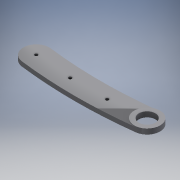
# Autodesk Inventor part: Arm 16X
Saved by Autodesk Inventor 2017 (Build 210142000, 142)
## iProperties
Created: 2016-03-22
Part Number: Arm 16X
Material: Generic
Document SubType Name: Modeling
Designer: alist
Density: 1 g/cm^3
Appearance: Default
Author: alist
Autodesk Inventor part; units mm, degrees
ref_plane "YZ Plane" through (0, 0, 0) normal (1, 0, 0) x (0, 1, 0)
ref_plane "XZ Plane" through (0, 0, 0) normal (0, 1, 0) x (-1, 0, 0)
ref_plane "XY Plane" through (0, 0, 0) normal (0, 0, 1) x (1, 0, 0)
sketch "Sketch1" plane through (0, 0, 0) normal (0, 0, 1) x (1, 0, 0)
  arc A0 (-74.2, 0) -> (74.2, 0) centre (0, 603.0231) ccw construction
  arc A1 (-76.3128, -17.1705) -> (76.3128, -17.1705) centre (0, 603.0231) ccw
  arc A2 (-72.0872, 17.1705) -> (72.0872, 17.1705) centre (0, 603.0231) ccw
  arc A3 (-72.0872, 17.1705) -> (-76.3128, -17.1705) centre (-74.2, 0) ccw
  arc A4 (76.3128, -17.1705) -> (72.0872, 17.1705) centre (74.2, 0) ccw
  line L0 (-159.9202, 0) -> (186.0645, 0) construction
  line L1 (0, 827.4607) -> (0, -503.7998) construction
  line L2 (74.2, 0) -> (74.2, 0) construction
  line L3 (74.2, 0) -> (91.3705, 2.1128) construction
  line L4 (74.2, 0) -> (72.0872, 17.1705) construction
  circle A5 centre (-74.2, 0) radius 2.15
  circle A6 centre (-24.7333, -4.0442) radius 2.15
  circle A7 centre (24.7333, -4.0442) radius 2.15
  circle A8 centre (74.2, 0) radius 11
  point P0 (0, 0)
  dimension "d0" = 148.4
  dimension "d1" = 34.6
  dimension "d2" = 603.0231
  dimension "d6" = 49.4667
  dimension "d7" = 24.7333
  dimension "d8" = 4.3
  dimension "d9" = 4.3
  dimension "d10" = 4.3
  dimension "d12" = 22
  constraints: 14 point on circle, 10 end point, 9 centre point, 6 tangent, 5 coincident, 5 point on line, 1 horizontal, 1 perpendicular, 1 vertical
  measures "d0" distance of A0.start L2.start
  measures "d1" diameter of A4
  measures "d2" distance from line of A0.centre L0
  measures "d6" distance of point (24.733, -4.044) point (-24.733, -4.044)
  measures "d7" horizontal distance of point (24.733, -4.044) point (0, 0)
  measures "d8" diameter of A5
  measures "d9" diameter of A6
  measures "d10" diameter of A7
  measures "d12" diameter of A8
extrude "Extrusion1" add sketch "Sketch1" along normal blind 6
sketch "Sketch2" plane through (0, 0, 6) normal (0, 0, 1) x (1, 0, 0)
  circle A0 centre (74.2, 0) radius 11 projected
  arc A1 (76.3128, -17.1705) -> (72.0872, 17.1705) centre (74.2, 0) ccw projected
  arc A2 (-76.3128, -17.1705) -> (76.3128, -17.1705) centre (0, 603.0231) ccw projected
  circle A3 centre (74.2, 0) radius 17.3
  point P0 (0, 0)
  constraints: 1 coincident, 3 other
extrude "Extrusion2" add sketch "Sketch2" along normal blind 1
sketch "Sketch3" plane through (0, 0, 0) normal (0, 0, -1) x (-1, 0, 0)
  circle A0 centre (-24.7333, -4.0442) radius 2.15 projected
  circle A1 centre (-24.7333, -4.0442) radius 3.95
  circle A2 centre (24.7333, -4.0442) radius 2.15 projected
  circle A3 centre (24.7333, -4.0442) radius 3.95
  point P0 (0, 0)
  dimension "d19" = 7.9
  dimension "d20" = 7.9
  constraints: 2 centre point, 2 coincident
  measures "d19" diameter of A1
  measures "d20" diameter of A3
extrude "Extrusion3" cut sketch "Sketch3" against normal blind 3
chamfer "Chamfer1" distance 1.8 angle 45 2 edges at (22.5833, -4.0442, 3) (-26.8833, -4.0442, 3)
equation "\"d6\" = 0.333333 * d0"
equation "\"d7\" = 0.5 * d6"
equation "\"d20\" = d19"
body "Solid1"
